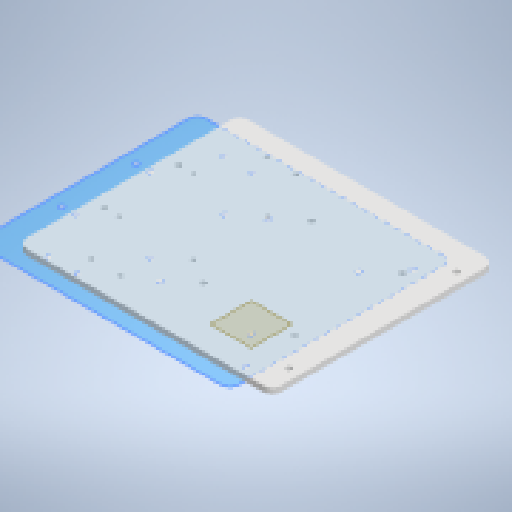
# Autodesk Inventor part: Top base 2
Saved by Autodesk Inventor 2023 (Build 270158000, 158)
## iProperties
Created: 2024-10-04
Part Number: Top base 2
Material: Generic
Document SubType Name: Modeling
Designer: bw1293
Density: 1 g/cm^3
Appearance: Default
Author: bw1293
Autodesk Inventor part; units mm, degrees
ref_plane "YZ Plane" through (0, 0, 0) normal (1, 0, 0) x (0, 1, 0)
ref_plane "XZ Plane" through (0, 0, 0) normal (0, 1, 0) x (-1, 0, 0)
ref_plane "XY Plane" through (0, 0, 0) normal (0, 0, 1) x (1, 0, 0)
sketch "Sketch1" plane through (0, 0, 0) normal (0, 1, 0) x (-1, 0, 0)
  line L0 (-31.6431, 25.3606) -> (38.3569, 25.3606)
  line L1 (100.8569, -14.6394) -> (100.8569, -54.6394)
  line L2 (-31.6431, -94.6394) -> (38.3569, -94.6394)
  arc A0 (-36.6431, -89.6394) -> (-31.6431, -94.6394) centre (-31.6431, -89.6394) ccw
  line L3 (-36.6431, -89.6394) -> (-36.6431, 20.3606)
  arc A1 (-31.6431, 25.3606) -> (-36.6431, 20.3606) centre (-31.6431, 20.3606) ccw
  circle A2 centre (-30.6431, 10.3606) radius 1.5
  circle A3 centre (45.8569, -54.6394) radius 1.25
  circle A4 centre (45.8569, -14.6394) radius 1.25
  circle A5 centre (85.8569, -14.6394) radius 1.25
  circle A6 centre (93.8569, -14.6394) radius 1.5
  circle A7 centre (93.8569, -54.6394) radius 1.5
  circle A8 centre (85.8569, -54.6394) radius 1.25
  circle A9 centre (-30.6431, -79.6394) radius 1.5
  line L4 (38.3569, -94.6394) -> (95.8569, -94.6394)
  line L5 (100.8569, -89.6394) -> (100.8569, 20.3606)
  line L6 (95.8569, 25.3606) -> (38.3569, 25.3606)
  arc A10 (95.8569, -94.6394) -> (100.8569, -89.6394) centre (95.8569, -89.6394) ccw
  arc A11 (100.8569, 20.3606) -> (95.8569, 25.3606) centre (95.8569, 20.3606) ccw
  line L7 (45.8569, -89.6394) -> (60.8569, -89.6394)
  line L8 (60.8569, -89.6394) -> (60.8569, -79.0394)
  line L9 (60.8569, -79.0394) -> (45.8569, -79.0394)
  line L10 (45.8569, -79.0394) -> (45.8569, -89.6394)
  line L11 (85.8569, -89.6394) -> (70.8569, -89.6394)
  line L12 (70.8569, -89.6394) -> (70.8569, -79.0394)
  line L13 (70.8569, -79.0394) -> (85.8569, -79.0394)
  line L14 (85.8569, -79.0394) -> (85.8569, -89.6394)
  line L15 (45.8569, 25.3606) -> (45.8569, 20.3606)
  line L16 (45.8569, 20.3606) -> (60.8569, 20.3606)
  line L17 (60.8569, 20.3606) -> (60.8569, 9.7606)
  line L18 (60.8569, 9.7606) -> (45.8569, 9.7606)
  line L19 (45.8569, 9.7606) -> (45.8569, 20.3606)
  line L20 (85.8569, 20.3606) -> (70.8569, 20.3606)
  line L21 (70.8569, 20.3606) -> (70.8569, 9.7606)
  line L22 (70.8569, 9.7606) -> (85.8569, 9.7606)
  line L23 (85.8569, 9.7606) -> (85.8569, 20.3606)
  line L24 (60.8569, -79.0394) -> (58.0285, -81.8678)
  line L25 (60.8569, -79.0394) -> (64.8569, -79.0394) construction
  line L26 (70.8569, -79.0394) -> (73.6853, -81.8678)
  line L27 (60.8569, 9.7606) -> (58.0285, 12.589)
  line L28 (60.8569, 9.7606) -> (64.8569, 9.7606) construction
  line L29 (70.8569, 9.7606) -> (73.6853, 12.589)
  line L30 (70.8569, 9.7606) -> (74.8569, 9.7606) construction
  circle A12 centre (58.0285, 12.589) radius 1.25
  circle A13 centre (73.6853, 12.589) radius 1.25
  circle A14 centre (73.6853, -81.8678) radius 1.25
  circle A15 centre (58.0285, -81.8678) radius 1.25
  point P0 (0, 0)
  point P1 (-36.6431, -94.6394)
  point P2 (-36.6431, -94.6394)
  point P3 (-36.6431, -94.6394)
  point P4 (100.8569, 25.3606)
  dimension "d8" = 5
  dimension "d9" = 15
  dimension "d10" = 10.6
  dimension "d11" = 15
  dimension "d12" = 10.6
  dimension "d13" = 5
  dimension "d14" = 5
  dimension "d15" = 15
  dimension "d16" = 10.6
  dimension "d17" = 15
  dimension "d18" = 10.6
  dimension "d19" = 4
  dimension "d20" = 135
  dimension "d21" = 4
  dimension "d22" = 4
  dimension "d23" = 135
  dimension "d24" = 4
  dimension "d25" = 45
  dimension "d26" = 2.5
  dimension "d27" = 2.5
  dimension "d28" = 2.5
  dimension "d29" = 2.5
  constraints: 62 end point, 16 centre point, 10 horizontal, 8 parallel, 8 point on circle, 5 perpendicular, 5 point on line, 4 coincident, 4 tangent, 3 equal length, 3 vertical, 1 equal radius, 32 other
  measures "d8" radius of A10
  measures "d9" distance of L9.end L8.end
  measures "d10" distance of L8.end L7.end
  measures "d11" distance of L12.end L13.end
  measures "d12" distance of L11.end L12.end
  measures "d13" distance between parallel lines of L4 L7
  measures "d14" distance of L15.start L15.end
  measures "d15" distance of L17.end L18.end
  measures "d16" distance of L16.end L17.end
  measures "d17" distance of L22.end L21.end
  measures "d18" distance of L21.end L20.end
  measures "d19" distance of L8.end L24.end
  measures "d20" angle of L24 L25
  measures "d21" distance of L12.end L26.end
  measures "d22" distance of L17.end L27.end
  measures "d23" angle of L28 L27
  measures "d24" distance of L21.end L29.end
  measures "d25" angle of L30 L29
  measures "d26" diameter of A12
  measures "d27" diameter of A13
  measures "d28" diameter of A14
  measures "d29" diameter of A15
ref_plane "Work Plane1" through (0, 3, 0) normal (0, 1, 0) x (1, 0, 0)
sketch "Sketch2" plane through (0, 3, 0) normal (0, 1, 0) x (1, 0, 0)
  circle A0 centre (16.7477, 6.3332) radius 1.25 projected
  circle A1 centre (-32.2523, 6.3332) radius 1.25 projected
  circle A2 centre (-32.2523, 64.3332) radius 1.25 projected
  circle A3 centre (16.7477, 64.3332) radius 1.25 projected
  circle A4 centre (16.7477, 64.3332) radius 1.5
  circle A5 centre (-32.2523, 64.3332) radius 1.5
  circle A6 centre (-32.2523, 6.3332) radius 1.5
  circle A7 centre (16.7477, 6.3332) radius 1.5
  point P0 (0, 0)
  dimension "d2" = 3
  dimension "d3" = 3
  dimension "d4" = 3
  dimension "d5" = 3
  constraints: 4 centre point, 4 coincident
  measures "d2" diameter of A4
  measures "d3" diameter of A5
  measures "d4" diameter of A6
  measures "d5" diameter of A7
extrude "Extrusion3" add sketch "Sketch1" along normal blind 3 contours L0 L6 A11 L5 L1 A10 L4 L2 A0 L3 A1 | L10 L9 L8 L7 | L11 L12 L13 L14 | L16 L17 L18 L19 | L23 L22 L21 L20
extrude "Extrusion4" cut sketch "Sketch2" against normal blind 3 contours A0 | A1 | A2 | A3 | A4 | A5 | A6 | A7
body "Solid2"
